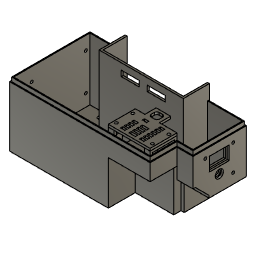
electronics_case (Autodesk Fusion 360 design; units mm, degrees)
Autodesk Fusion 360 part; units mm, degrees
(part 1 of 2)
sketch "Bodenplatte" plane through (0, 0, 0) normal (0, 0, 1) x (1, 0, 0) in component "Boden"
  line L0 (0, 0) -> (123, 0)
  line L1 (175, 42.5) -> (175, 80)
  line L2 (154, 100) -> (0, 100)
  line L3 (0, 100) -> (0, 0)
  line L4 (171, 33.5) -> (123, 33.5)
  line L5 (123, 33.5) -> (123, 0)
  line L6 (154, 100) -> (154, 80)
  line L7 (154, 80) -> (175, 80)
  line L8 (175, 42.5) -> (171, 42.5)
  line L9 (171, 42.5) -> (171, 33.5)
  line L10 (120.5, 20) -> (105.5, 20)
  line L11 (105.5, 20) -> (105.5, 35)
  line L12 (105.5, 35) -> (120.5, 35)
  line L13 (120.5, 35) -> (120.5, 20)
  dimension "d2" = 100
  dimension "d3" = 20
  dimension "d4" = 21
  dimension "d7" = 33
  dimension "d8" = 4
  dimension "d9" = 9
  dimension "d10" = 49
  dimension "d11" = 133.3838
  dimension "d12" = 15
  dimension "d13" = 15
  dimension "d14" = 2.5
  dimension "d76" = 37.5
  dimension "d77" = 52
  dimension "d83" = 20
  dimension "d153" = 175
  constraint horizontal L0
  constraint vertical L1
  constraint horizontal L2
  constraint vertical L3
  constraint coincident L0.start L3.end
  constraint perpendicular L1 L4
  constraint perpendicular L0 L5
  constraint perpendicular L2 L6
  constraint perpendicular L1 L7
  constraint perpendicular L1 L8
  constraint perpendicular L4 L9
  constraint horizontal L10
  constraint vertical L11
  constraint horizontal L12
  constraint vertical L13
  measures "d2" distance of L0.start L2.end
  measures "d3" distance of L2.start L6.end
  measures "d4" distance of L6.end L1.end
  measures "d8" distance of L1.start L8.end
  measures "d9" distance of L8.end L4.start
  measures "d12" distance of L10.start L10.end
  measures "d13" distance of L10.start L12.end
  measures "d14" distance of L5 L13
  measures "d76" distance of L1.end L1.start
  measures "d77" distance of L1 L5
  measures "d83" distance of L0 L10
  measures "d153" distance of L1 L3
extrude "Extrude1" add sketch "Bodenplatte" along normal blind 2.5 makes body 1 in component "Boden"
sketch "Winkel" plane through (0, 100, 0) normal (0, 1, 0) x (-1, 0, 0) in component "Boden"
  line L0 (-154, 0) -> (0, 0)
  line L1 (0, 0) -> (0, 2.5)
  line L2 (0, 2.5) -> (-154, 2.5)
  line L3 (-154, 2.5) -> (-154, 0)
  line L4 (-154, 2.5) -> (-154, 3.5)
  line L5 (-154, 3.5) -> (-170.5, 20)
  line L6 (-170.5, 20) -> (-195, 20)
  line L7 (-195, 20) -> (-195, 22.5)
  line L8 (-195, 22.5) -> (-169.4645, 22.5)
  line L9 (-169.4645, 22.5) -> (-151.5, 4.5355)
  line L10 (-151.5, 4.5355) -> (-151.5, 2.5)
  line L11 (-175, 0) -> (-175, 2.5)
  line L12 (-123, 2.5) -> (-171, 2.5)
  line L13 (-154, 0) -> (0, 0)
  dimension "d17" = 135
  dimension "d19" = 20.5
  dimension "d20" = 2.5
  dimension "d21" = 2.5
  dimension "d22" = 2.5
  dimension "d24" = 20
  dimension "d44" = 3.5
  dimension "d45" = 4.5
  constraint coincident L2.end L3.start
  constraint perpendicular L2 L4
  constraint horizontal L6
  constraint perpendicular L6 L7
  constraint perpendicular L7 L8
  constraint parallel L5 L9
  constraint coincident L2 L10.end
  constraint perpendicular L2 L10
  measures "d17" angle of L4 L5
  measures "d20" distance of L6.end L7.end
  measures "d21" distance of L5 L9
  measures "d22" distance of L4 L10
  measures "d24" distance of L7 L11
  measures "d44" distance of L4.end L13
  measures "d45" distance of L5.end L11
extrude "Extrude6" add sketch "Winkel" against normal up to surface (20 mm away) contours L2 L4 L5 L6 L7 L8 L9 L10 L12 bodies 1 in component "Boden"
sketch "Winkelabdeckung" plane through (0, 80, 0) normal (0, -1, 0) x (1, 0, 0) in component "Boden"
  line L0 (195, 22.5) -> (169.4645, 22.5)
  line L1 (169.4645, 22.5) -> (151.5, 4.5355)
  line L2 (151.5, 4.5355) -> (151.5, 2.5)
  line L3 (151.5, 2.5) -> (154, 2.5)
  line L4 (154, 2.5) -> (154, 3.5) construction
  line L5 (154, 3.5) -> (170.5, 20) construction
  line L6 (170.5, 20) -> (195, 20) construction
  line L7 (195, 20) -> (195, 22.5)
  line L8 (151.5, 2.5) -> (151.5, 4.5355)
  line L9 (151.5, 4.5355) -> (169.4645, 22.5)
  line L10 (186.3838, 2.5) -> (151.5, 2.5)
  line L11 (175, 0) -> (175, 2.5)
  line L12 (175, 2.5) -> (175, 20)
  line L13 (175, 20) -> (195, 20)
  line L14 (195, 20) -> (195, 22.5)
  line L15 (195, 22.5) -> (169.4645, 22.5)
  constraint coincident L2.end L3.start
  constraint coincident L1.end L2.start
  constraint coincident L0.end L1.start
  constraint perpendicular L8 L10
  constraint coincident L11.end L12.start
  constraint coincident L6 L12.end
  constraint perpendicular L6 L12
  constraint coincident L6.end L7.start
  constraint coincident L0.start L7.end
extrude "Extrude7" add sketch "Winkelabdeckung" along normal blind 2.5 bodies 1 in component "Boden"
sketch "Stangenabdeckung" plane through (0, 77.5, 0) normal (0, -1, 0) x (1, 0, 0) in component "Boden"
  line L0 (175, 2.5) -> (175, 20)
  line L1 (175, 20) -> (195, 20)
  line L2 (195, 20) -> (195, 22.5)
  line L3 (195, 22.5) -> (169.4645, 22.5)
  line L4 (169.4645, 22.5) -> (151.5, 4.5355)
  line L5 (151.5, 4.5355) -> (151.5, 2.5)
  line L6 (151.5, 2.5) -> (175, 2.5)
  line L7 (175, 20) -> (195, 20)
  line L8 (195, 20) -> (195, 22.5)
  line L9 (195, 22.5) -> (172.5, 22.5)
  line L10 (172.5, 22.5) -> (172.5, 2.5)
  line L11 (172.5, 2.5) -> (175, 2.5)
  line L12 (175, 2.5) -> (175, 20)
  dimension "d50" = 2.5
  constraint coincident L0.end L1.start
  constraint coincident L1.end L2.start
  constraint coincident L2.end L3.start
  constraint coincident L3 L9.end
  constraint perpendicular L8 L9
  constraint coincident L6 L10.end
  constraint perpendicular L6 L10
  constraint coincident L0.start L6.end
  measures "d50" distance of L10 L12
extrude "Extrude8" add sketch "Stangenabdeckung" along normal blind 26.5 from surface at -2.5 contours L0 L1 L2 L3 L6 L7 L8 L9 L10 L11 L12 bodies 1 in component "Boden"
sketch "Seitenwinkel" plane through (195, 0, 0) normal (1, 0, 0) x (0, 1, 0) in component "Boden"
  line L0 (53.5, 20) -> (100, 20)
  line L1 (100, 20) -> (100, 22.5)
  line L2 (100, 22.5) -> (53.5, 22.5)
  line L3 (53.5, 22.5) -> (53.5, 20)
  line L4 (53.5, 22.5) -> (53.5, 23)
  line L5 (53.5, 23) -> (36.5, 40)
  line L6 (37.5355, 42.5) -> (56, 24.0355)
  line L7 (56, 24.0355) -> (56, 22.5)
  line L8 (36.5, 40) -> (33.5, 40)
  line L9 (33.5, 40) -> (33.5, 42.5)
  line L10 (33.5, 42.5) -> (37.5355, 42.5)
  dimension "d54" = 135
  dimension "d56" = 2.5
  dimension "d57" = 2.5
  dimension "d58" = 2.5
  dimension "d60" = 3
  dimension "d61" = 3
  dimension "d62" = 20
  dimension "d63" = 20
  constraint coincident L2.end L3.start
  constraint perpendicular L2 L4
  constraint parallel L5 L6
  constraint coincident L2 L7.end
  constraint perpendicular L2 L7
  constraint horizontal L8
  constraint perpendicular L8 L9
  constraint perpendicular L9 L10
  measures "d54" angle of L4 L5
  measures "d56" distance of L4 L7
  measures "d57" distance of L5 L6
  measures "d58" distance of L8.end L9.end
  measures "d60" distance of L5.end L8.end
  measures "d61" distance of L0 L4.end
  measures "d62" distance of L3 L9
  measures "d63" distance of L0 L8
extrude "Extrude9" add sketch "Seitenwinkel" against normal up to surface (20 mm away) contours L2 L4 L5 L6 L7 L8 L9 L10 bodies 1 in component "Boden"
sketch "Seitenwinkelabdeckung" plane through (175, 0, 0) normal (1, 0, 0) x (0, 1, 0) in component "Boden"
  line L0 (53.5, 2.5) -> (42.5, 2.5)
  line L1 (42.5, 2.5) -> (42.5, 0)
  line L2 (42.5, 0) -> (80, 0)
  line L3 (80, 0) -> (80, 20)
  line L4 (80, 20) -> (53.5, 20)
  line L5 (53.5, 20) -> (53.5, 2.5)
  line L6 (45, 2.5) -> (53.5, 2.5)
  line L7 (45, 35.0355) -> (45, 2.5)
  line L8 (53.5, 23) -> (36.5, 40)
  line L9 (37.5355, 42.5) -> (56, 24.0355)
  line L10 (53.5, 2.5) -> (53.5, 22.5)
  line L11 (53.5, 22.5) -> (56, 22.5)
  line L12 (56, 22.5) -> (56, 24.0355)
  line L13 (56, 24.0355) -> (45, 35.0355)
  line L14 (56, 24.0355) -> (56, 22.5)
  line L15 (77.5, 22.5) -> (53.5, 22.5)
  dimension "d66" = 4
  dimension "d70" = 2.5
  constraint coincident L0.start L5.end
  constraint perpendicular L6 L7
  constraint perpendicular L6 L10
  constraint perpendicular L10 L11
  constraint collinear L9 L13
  constraint collinear L12 L14
  constraint collinear L11 L15
  measures "d70" distance of L1 L7
extrude "Extrude10" add sketch "Seitenwinkelabdeckung" against normal up to surface (2.5 mm away) contours L0 L5 L6 L7 L9 L10 L11 L12 L13 L14 L15 bodies 1 in component "Boden"
sketch "Sketch8" plane through (0, 0, 2.5) normal (0, 0, 1) x (-1, 0, 0) in component "Boden"
  line L0 (-105.5, -35) -> (-120.5, -35)
  line L1 (-120.5, -35) -> (-120.5, -20)
  line L2 (-120.5, -20) -> (-105.5, -20)
  line L3 (-105.5, -20) -> (-105.5, -35)
  line L4 (-175, -45) -> (-172.5, -45)
  line L5 (-172.5, -45) -> (-172.5, -77.5)
  line L6 (-172.5, -77.5) -> (-151.5, -77.5)
  line L7 (-151.5, -77.5) -> (-151.5, -100)
  line L8 (-151.5, -100) -> (0, -100)
  line L9 (0, -100) -> (0, 0)
  line L10 (0, 0) -> (-123, 0)
  line L11 (-123, 0) -> (-123, -33.5)
  line L12 (-123, -33.5) -> (-171, -33.5)
  line L13 (-171, -33.5) -> (-171, -42.5)
  line L14 (-171, -42.5) -> (-175, -42.5)
  line L15 (-175, -42.5) -> (-175, -45)
  line L16 (-172.5, -45) -> (-168.5, -45)
  line L17 (-168.5, -45) -> (-168.5, -33.5)
  dimension "d71" = 2.5
  constraint coincident L4.end L5.start
  constraint perpendicular L5 L16
  constraint coincident L12 L17.end
  constraint perpendicular L12 L17
  measures "d71" distance of L13 L17
extrude "Extrude11" add sketch "Sketch8" along normal up to surface (52 mm away) contours L4 L12 L13 L14 L15 L16 L17 bodies 1 in component "Boden"
sketch "Sketch9" plane through (175, 0, 0) normal (-1, 0, 0) x (0, -1, 0) in component "Boden"
  line L0 (-42.5, 37.5355) -> (-42.5, 34)
  line L1 (-42.5, 34) -> (-36.5, 40)
  line L2 (-36.5, 40) -> (-33.5, 40)
  line L3 (-33.5, 40) -> (-33.5, 42.5)
  line L4 (-33.5, 42.5) -> (-37.5355, 42.5)
  line L5 (-37.5355, 42.5) -> (-42.5, 37.5355)
  line L6 (-45, 35.0355) -> (-45, 54.5)
  line L7 (-45, 54.5) -> (-33.5, 54.5)
  line L8 (-33.5, 54.5) -> (-33.5, 42.5)
  line L9 (-37.5355, 42.5) -> (-45, 35.0355)
  line L10 (-45, 35.0355) -> (-45, 54.5)
  line L11 (-33.5, 42.5) -> (-37.5355, 42.5)
  line L12 (-45, 54.5) -> (-42.5, 54.5)
  constraint vertical L6
  constraint perpendicular L6 L7
  constraint coincident L4 L3.end
  constraint perpendicular L4 L8
  constraint coincident L4.end L5.start
  constraint collinear L3 L8
  constraint collinear L6 L10
  constraint collinear L5 L9
  constraint collinear L7 L12
extrude "Extrude12" add sketch "Sketch9" against normal blind 2.5 contours L4 L5 L6 L7 L8 L9 L10 L11 L12 bodies 1 in component "Boden"
sketch "Sketch11" plane through (0, 0, 42.5) normal (0, 0, 1) x (-1, 0, 0) in component "Boden"
  line L0 (-177.5, -37.5355) -> (-177.5, -33.5)
  line L1 (-177.5, -33.5) -> (-195, -33.5)
  line L2 (-195, -33.5) -> (-195, -37.5355)
  line L3 (-195, -37.5355) -> (-177.5, -37.5355)
  line L4 (-177.5, -33.5) -> (-195, -33.5)
  line L5 (-195, -33.5) -> (-195, -36)
  line L6 (-195, -36) -> (-177.5, -36)
  line L7 (-177.5, -36) -> (-177.5, -33.5)
  dimension "d78" = 2.5
  constraint horizontal L4
  constraint vertical L5
  constraint horizontal L6
  constraint vertical L7
  constraint coincident L2 L5.end
  constraint coincident L0.end L1.start
  measures "d78" distance of L1.end L5.end
extrude "Extrude13" add sketch "Sketch11" along normal up to surface (12 mm away) contours L0 L1 L2 L4 L5 L6 L7 bodies 1 in component "Boden"
sketch "Sketch12" plane through (195, 0, 0) normal (1, 0, 0) x (0, 1, 0) in component "Boden"
  line L0 (53.5, 20) -> (100, 20)
  line L1 (100, 20) -> (100, 22.5)
  line L2 (100, 22.5) -> (56, 22.5)
  line L3 (56, 22.5) -> (56, 24.0355)
  line L4 (56, 24.0355) -> (37.5355, 42.5)
  line L5 (37.5355, 42.5) -> (36, 42.5)
  line L6 (36, 42.5) -> (36, 54.5)
  line L7 (36, 54.5) -> (33.5, 54.5)
  line L8 (33.5, 54.5) -> (33.5, 40)
  line L9 (33.5, 40) -> (36.5, 40)
  line L10 (36.5, 40) -> (53.5, 23)
  line L11 (53.5, 23) -> (53.5, 20)
  line L12 (100, 22.5) -> (56, 22.5)
  line L13 (56, 24.0355) -> (37.5355, 42.5)
  line L14 (36, 42.5) -> (36, 54.5)
  line L15 (37.5355, 42.5) -> (36, 42.5)
  line L16 (36, 54.5) -> (100, 54.5)
  line L17 (100, 54.5) -> (100, 22.5)
  constraint coincident L1.end L2.start
  constraint coincident L2.end L3.start
  constraint coincident L3.end L4.start
  constraint coincident L4.end L5.start
  constraint coincident L5.end L6.start
  constraint coincident L6.end L7.start
  constraint perpendicular L14 L16
  constraint perpendicular L16 L17
extrude "Extrude14" add sketch "Sketch12" against normal blind 2.5 contours L2 L3 L4 L5 L6 L12 L13 L14 L15 L16 L17 bodies 1 in component "Boden"
sketch "Sketch13" plane through (0, 0, 2.5) normal (0, 0, 1) x (-1, 0, 0) in component "Boden"
  line L0 (-168.5, -33.5) -> (-168.5, -45)
  line L1 (-168.5, -45) -> (-172.5, -45)
  line L2 (-172.5, -45) -> (-172.5, -77.5)
  line L3 (-172.5, -77.5) -> (-151.5, -77.5)
  line L4 (-151.5, -77.5) -> (-151.5, -100)
  line L5 (-151.5, -100) -> (0, -100)
  line L6 (0, -100) -> (0, 0)
  line L7 (0, 0) -> (-123, 0)
  line L8 (-123, 0) -> (-123, -33.5)
  line L9 (-123, -33.5) -> (-168.5, -33.5)
  line L10 (-105.5, -35) -> (-120.5, -35)
  line L11 (-120.5, -35) -> (-120.5, -20)
  line L12 (-120.5, -20) -> (-105.5, -20)
  line L13 (-105.5, -20) -> (-105.5, -35)
  line L14 (-168.5, -36) -> (-120.5, -36)
  line L15 (-120.5, -36) -> (-120.5, -20)
  line L16 (-120.5, -20) -> (-105.5, -20)
  line L17 (-105.5, -20) -> (-105.5, -35)
  line L18 (-105.5, -35) -> (-103, -35)
  line L19 (-103, -35) -> (-103, -17.5)
  line L20 (-103, -17.5) -> (-120.5, -17.5)
  line L21 (-120.5, -17.5) -> (-120.5, 0)
  line L22 (-192.5, -36) -> (-177.5, -36)
  dimension "d84" = 2.5
  dimension "d85" = 2.5
  constraint coincident L0 L14.start
  constraint perpendicular L0 L14
  constraint perpendicular L14 L15
  constraint perpendicular L15 L16
  constraint perpendicular L10 L17
  constraint perpendicular L17 L18
  constraint perpendicular L18 L19
  constraint perpendicular L19 L20
  constraint coincident L7 L21.end
  constraint perpendicular L7 L21
  constraint collinear L11 L15
  constraint collinear L12 L16
  constraint collinear L13 L17
  constraint collinear L10 L18
  constraint collinear L15 L21
  constraint collinear L14 L22
  measures "d84" distance of L17 L19
  measures "d85" distance of L16 L20
extrude "Extrude15" add sketch "Sketch13" along normal up to surface (52 mm away) contours L0 L7 L8 L9 L11 L12 L13 L14 L15 L16 L17 L18 L19 L20 L21 bodies 1 in component "Boden"
sketch "Sketch1" plane through (192.5, 0, 0) normal (-1, 0, 0) x (0, -1, 0) in component "Stromanschluss"
  line L0 (-36, 54.5) -> (-100, 54.5) construction
  line L1 (-100, 54.5) -> (-100, 22.5)
  line L2 (-100, 22.5) -> (-56, 22.5)
  line L3 (-56, 22.5) -> (-56, 24.0355)
  line L4 (-56, 24.0355) -> (-37.5355, 42.5)
  line L5 (-37.5355, 42.5) -> (-36, 42.5)
  line L6 (-36, 42.5) -> (-36, 54.5)
  line L7 (-76.6, 63) -> (-56, 63)
  line L8 (-56, 63) -> (-56, 50)
  line L9 (-56, 50) -> (-76.6, 50)
  line L10 (-76.6, 50) -> (-76.6, 63)
  circle A0 centre (-66.3, 39.75) radius 3.65
  circle A1 centre (-66.3, 39.75) radius 5.25
  line L11 (-76.6, 50) -> (-56, 63) construction
  line L12 (-76.6, 63) -> (-56, 50) construction
  line L13 (-88.6, 70) -> (-44, 70)
  line L14 (-44, 70) -> (-44, 42.5)
  line L15 (-59, 27.5) -> (-88.6, 27.5)
  line L16 (-88.6, 27.5) -> (-88.6, 70)
  line L17 (-59, 27.5) -> (-44, 42.5)
  circle A2 centre (-83.6, 32.5) radius 1.75
  circle A3 centre (-83.6, 65) radius 1.75
  circle A4 centre (-49, 65) radius 1.75
  point P0 (-66.3, 56.5)
  dimension "d91" = 20.6
  dimension "d92" = 13
  dimension "d93" = 7.3
  dimension "d94" = 10.5
  dimension "d95" = 5
  dimension "d96" = 7
  dimension "d97" = 7
  dimension "d98" = 12
  dimension "d99" = 12
  dimension "d105" = 135
  dimension "d106" = 15
  dimension "d107" = 5
  dimension "d108" = 8
  dimension "d113" = 3.5
  dimension "d114" = 5
  dimension "d115" = 5
  dimension "d116" = 5
  dimension "d117" = 5
  constraint horizontal L7
  constraint vertical L8
  constraint horizontal L9
  constraint vertical L10
  constraint concentric A0 A1
  constraint midpoint L12 P0
  constraint vertical A0.centre P0
  constraint horizontal L13
  constraint vertical L14
  constraint horizontal L15
  constraint vertical L16
  constraint vertical A2.centre A3.centre
  constraint horizontal A3.centre A4.centre
  constraint equal A2 A3
  constraint equal A2 A4
  measures "d91" distance of L7.start L7.end
  measures "d92" distance of L7.start L9.end
  measures "d93" diameter of A0
  measures "d94" diameter of A1
  measures "d95" distance of L9 A1
  measures "d96" distance of A1 L15
  measures "d97" distance of L7 L13
  measures "d98" distance of L10 L16
  measures "d99" distance of L8 L14
  measures "d105" angle of L15 L17
  measures "d106" vertical distance of L15.start L14.end
  measures "d107" distance of L2 L15
  measures "d108" distance of L6 L14
  measures "d113" diameter of A2
  measures "d114" distance of L15 A2.centre
  measures "d115" distance of L16 A2.centre
  measures "d116" distance of L13 A3.centre
  measures "d117" distance of L14 A4.centre
sketch "Sketch15" plane through (0, 100, 0) normal (0, 1, 0) x (-1, 0, 0) in component "Boden"
  line L0 (-154, 0) -> (0, 0)
  line L1 (0, 0) -> (0, 2.5)
  line L2 (0, 2.5) -> (-151.5, 2.5)
  line L3 (-151.5, 2.5) -> (-151.5, 4.5355)
  line L4 (-151.5, 4.5355) -> (-169.4645, 22.5)
  line L5 (-169.4645, 22.5) -> (-192.5, 22.5)
  line L6 (-192.5, 22.5) -> (-192.5, 54.5)
  line L7 (-192.5, 54.5) -> (-195, 54.5)
  line L8 (-195, 54.5) -> (-195, 20)
  line L9 (-195, 20) -> (-170.5, 20)
  line L10 (-170.5, 20) -> (-154, 3.5)
  line L11 (-154, 3.5) -> (-154, 0)
  line L12 (-192.5, 54.5) -> (-192.5, 22.5)
  line L13 (-192.5, 22.5) -> (-169.4645, 22.5)
  line L14 (-169.4645, 22.5) -> (-151.5, 4.5355)
  line L15 (-151.5, 4.5355) -> (-151.5, 2.5)
  line L16 (-151.5, 2.5) -> (-146.5, 2.5)
  line L17 (-146.5, 2.5) -> (-146.5, 54.5)
  line L18 (-146.5, 54.5) -> (-192.5, 54.5)
  dimension "d102" = 5
  constraint coincident L6.end L7.start
  constraint coincident L5.end L6.start
  constraint coincident L4.end L5.start
  constraint coincident L3.end L4.start
  constraint coincident L2.end L3.start
  constraint coincident L2 L16.end
  constraint perpendicular L3 L16
  constraint perpendicular L16 L17
  constraint perpendicular L17 L18
  measures "d102" distance of L2.end L16.end
extrude "Extrude17" add sketch "Sketch15" against normal blind 2.5 contours L2 L3 L4 L5 L6 L12 L13 L14 L15 L16 L17 L18 bodies 1 in component "Boden"
extrude "Extrude1'" add sketch "Sketch1" along normal blind 2.5 separate body contours L13 L14 L15 L16 L17 makes body 2 in component "Stromanschluss"
extrude "Extrude2" add sketch "Sketch1" along normal blind 2 contours A1 bodies 2 in component "Stromanschluss"
sketch "Sketch17" plane through (0, 0, 54.5) normal (0, 0, 1) x (-1, 0, 0) in component "Boden"
  line L0 (-177.5, -45) -> (-168.5, -45)
  line L1 (-168.5, -45) -> (-168.5, -36)
  line L2 (-168.5, -36) -> (-120.5, -36)
  line L3 (-120.5, -36) -> (-120.5, -20)
  line L4 (-120.5, -20) -> (-105.5, -20)
  line L5 (-105.5, -20) -> (-105.5, -35)
  line L6 (-105.5, -35) -> (-103, -35)
  line L7 (-103, -35) -> (-103, -17.5)
  line L8 (-103, -17.5) -> (-120.5, -17.5)
  line L9 (-120.5, -17.5) -> (-120.5, 0)
  line L10 (-120.5, 0) -> (-123, 0)
  line L11 (-123, 0) -> (-123, -33.5)
  line L12 (-123, -33.5) -> (-171, -33.5)
  line L13 (-171, -33.5) -> (-171, -42.5)
  line L14 (-171, -42.5) -> (-175, -42.5)
  line L15 (-175, -42.5) -> (-175, -33.5)
  line L16 (-175, -33.5) -> (-195, -33.5)
  line L17 (-195, -33.5) -> (-195, -100)
  line L18 (-195, -100) -> (-146.5, -100)
  line L19 (-146.5, -100) -> (-146.5, -97.5)
  line L20 (-146.5, -97.5) -> (-192.5, -97.5)
  line L21 (-192.5, -97.5) -> (-192.5, -36)
  line L22 (-192.5, -36) -> (-177.5, -36)
  line L23 (-177.5, -36) -> (-177.5, -45)
  line L24 (-123, 0) -> (-175, 0)
  line L25 (-175, 0) -> (-175, -33.5)
  constraint coincident L10.end L11.start
  constraint perpendicular L11 L24
  constraint coincident L12 L15.end
  constraint perpendicular L12 L25
  constraint collinear L15 L25
extrude "Extrude18" add sketch "Sketch17" along normal blind 2.5 bodies 1 in component "Boden"
sketch "Sketch18" plane through (0, 0, 2.5) normal (0, 0, 1) x (-1, 0, 0) in component "Boden"
  line L0 (-146.5, -97.5) -> (-146.5, -100)
  line L1 (-146.5, -100) -> (0, -100)
  line L2 (0, -100) -> (0, 0)
  line L3 (0, 0) -> (-120.5, 0)
  line L4 (-120.5, 0) -> (-120.5, -17.5)
  line L5 (-120.5, -17.5) -> (-103, -17.5)
  line L6 (-103, -17.5) -> (-103, -35)
  line L7 (-103, -35) -> (-105.5, -35)
  line L8 (-105.5, -35) -> (-120.5, -35)
  line L9 (-120.5, -35) -> (-120.5, -36)
  line L10 (-120.5, -36) -> (-168.5, -36)
  line L11 (-168.5, -36) -> (-168.5, -45)
  line L12 (-168.5, -45) -> (-172.5, -45)
  line L13 (-172.5, -45) -> (-172.5, -77.5)
  line L14 (-172.5, -77.5) -> (-151.5, -77.5)
  line L15 (-151.5, -77.5) -> (-151.5, -97.5)
  line L16 (-151.5, -97.5) -> (-146.5, -97.5)
  line L17 (-163.5, -41) -> (-153.5, -41)
  line L18 (-153.5, -41) -> (-153.5, -51)
  line L19 (-153.5, -51) -> (-163.5, -51)
  line L20 (-163.5, -51) -> (-163.5, -41)
  dimension "d120" = 10
  dimension "d121" = 10
  dimension "d122" = 5
  dimension "d123" = 5
  constraint horizontal L17
  constraint vertical L18
  constraint horizontal L19
  constraint vertical L20
  measures "d120" distance of L17.start L17.end
  measures "d121" distance of L17.start L19.end
  measures "d122" distance of L10 L17
  measures "d123" distance of L11 L20
extrude "Extrude19" cut sketch "Sketch18" against normal up to surface (2.5 mm away) contours L17 L18 L19 L20 bodies 1 in component "Boden"
sketch "Sketch19" plane through (0, 0, 2.5) normal (0, 0, 1) x (-1, 0, 0) in component "Boden"
  line L0 (-163.5, -51) -> (-163.5, -41)
  line L1 (-163.5, -41) -> (-153.5, -41)
  line L2 (-153.5, -41) -> (-153.5, -51)
  line L3 (-153.5, -51) -> (-163.5, -51)
  line L4 (-146.5, -97.5) -> (-146.5, -100)
  line L5 (-146.5, -100) -> (0, -100)
  line L6 (0, -100) -> (0, 0)
  line L7 (0, 0) -> (-120.5, 0)
  line L8 (-120.5, 0) -> (-120.5, -17.5)
  line L9 (-120.5, -17.5) -> (-103, -17.5)
  line L10 (-103, -17.5) -> (-103, -35)
  line L11 (-103, -35) -> (-105.5, -35)
  line L12 (-105.5, -35) -> (-120.5, -35)
  line L13 (-120.5, -35) -> (-120.5, -36)
  line L14 (-120.5, -36) -> (-168.5, -36)
  line L15 (-168.5, -36) -> (-168.5, -45)
  line L16 (-168.5, -45) -> (-172.5, -45)
  line L17 (-172.5, -45) -> (-172.5, -77.5)
  line L18 (-172.5, -77.5) -> (-151.5, -77.5)
  line L19 (-151.5, -77.5) -> (-151.5, -97.5)
  line L20 (-151.5, -97.5) -> (-146.5, -97.5)
  line L21 (-146.5, -97.5) -> (-146.5, -70)
  line L22 (-146.5, -70) -> (-46.5, -70)
  line L23 (-46.5, -70) -> (-46.5, -100)
  line L24 (-44, -100) -> (-44, -67.5)
  line L25 (-44, -67.5) -> (-149, -67.5)
  line L26 (-149, -67.5) -> (-149, -97.5)
  dimension "d126" = 2.5
  dimension "d127" = 2.5
  dimension "d128" = 2.5
  dimension "d129" = 30
  dimension "d130" = 100
  constraint coincident L4.start L20.end
  constraint perpendicular L20 L21
  constraint perpendicular L21 L22
  constraint coincident L5 L23.end
  constraint perpendicular L5 L23
  constraint coincident L5 L24.start
  constraint perpendicular L5 L24
  constraint perpendicular L24 L25
  constraint coincident L20 L26.end
  constraint perpendicular L20 L26
  measures "d126" distance of L21 L26
  measures "d127" distance of L22 L25
  measures "d128" distance of L23 L24
  measures "d129" distance of L22.end L23.end
  measures "d130" distance of L21.end L22.end
extrude "Extrude20" add sketch "Sketch19" along normal blind 5 contours L4 L5 L21 L22 L23 bodies 1 in component "Boden"
extrude "Extrude21" add sketch "Sketch19" along normal up to surface (54.5 mm away) contours L5 L20 L21 L22 L23 L24 L25 L26 bodies 1 in component "Boden"
sketch "Sketch20" plane through (0, 0, 2.5) normal (0, 0, 1) x (-1, 0, 0) in component "Boden"
  line L0 (-163.5, -51) -> (-163.5, -41)
  line L1 (-163.5, -41) -> (-153.5, -41)
  line L2 (-153.5, -41) -> (-153.5, -51)
  line L3 (-153.5, -51) -> (-163.5, -51)
  line L4 (-149, -97.5) -> (-149, -67.5)
  line L5 (-149, -67.5) -> (-44, -67.5)
  line L6 (-44, -67.5) -> (-44, -100)
  line L7 (-44, -100) -> (0, -100)
  line L8 (0, -100) -> (0, 0)
  line L9 (0, 0) -> (-120.5, 0)
  line L10 (-120.5, 0) -> (-120.5, -17.5)
  line L11 (-120.5, -17.5) -> (-103, -17.5)
  line L12 (-103, -17.5) -> (-103, -35)
  line L13 (-103, -35) -> (-105.5, -35)
  line L14 (-105.5, -35) -> (-120.5, -35)
  line L15 (-120.5, -35) -> (-120.5, -36)
  line L16 (-120.5, -36) -> (-168.5, -36)
  line L17 (-168.5, -36) -> (-168.5, -45)
  line L18 (-168.5, -45) -> (-172.5, -45)
  line L19 (-172.5, -45) -> (-172.5, -77.5)
  line L20 (-172.5, -77.5) -> (-151.5, -77.5)
  line L21 (-151.5, -77.5) -> (-151.5, -97.5)
  line L22 (-151.5, -97.5) -> (-149, -97.5)
  line L23 (-107, -17.5) -> (-107, -15.5)
  line L24 (-107, -15.5) -> (-103, -15.5)
  line L25 (-103, -15.5) -> (-103, -13)
  line L26 (-103, -13) -> (-109.5, -13)
  line L27 (-109.5, -13) -> (-109.5, -17.5)
  line L28 (-20, -13) -> (-20, -15.5)
  line L29 (-20, -15.5) -> (-16, -15.5)
  line L30 (-16, -15.5) -> (-16, -17.5)
  line L31 (-16, -17.5) -> (-20, -17.5)
  line L32 (-20, -17.5) -> (-20, -20)
  line L33 (-20, -20) -> (-13.5, -20)
  line L34 (-13.5, -20) -> (-13.5, -13)
  line L35 (-13.5, -13) -> (-20, -13)
  line L36 (-120.5, -20) -> (-105.5, -20)
  line L37 (-103, -15.5) -> (-103, -17.5)
  line L38 (-20, -15.5) -> (-20, -17.5)
  dimension "d135" = 2
  dimension "d136" = 2.5
  dimension "d137" = 2.5
  dimension "d138" = 4
  dimension "d139" = 91
  dimension "d140" = 2
  dimension "d141" = 4
  dimension "d142" = 2.5
  constraint coincident L11 L23.start
  constraint perpendicular L11 L23
  constraint perpendicular L23 L24
  constraint perpendicular L11 L25
  constraint perpendicular L25 L26
  constraint coincident L11 L27.end
  constraint perpendicular L11 L27
  constraint perpendicular L26 L28
  constraint perpendicular L28 L29
  constraint perpendicular L26 L30
  constraint perpendicular L28 L31
  constraint perpendicular L31 L32
  constraint perpendicular L32 L33
  constraint perpendicular L33 L34
  constraint perpendicular L34 L35
  constraint collinear L12 L25
  constraint collinear L11 L31
  constraint collinear L33 L36
  constraint collinear L26 L35
  constraint collinear L28 L32
  constraint coincident L11.end L12.start
  measures "d135" distance of L23.start L23.end
  measures "d136" distance of L24 L26
  measures "d137" distance of L23 L27
  measures "d138" distance of L12 L23
  measures "d139" distance of L23 L30
  measures "d140" distance of L29.end L30.end
  measures "d141" distance of L30.end L31.end
  measures "d142" distance of L30 L34
extrude "Extrude22" add sketch "Sketch20" along normal blind 2.5 contours L11 L23 L24 L25 L26 L27 | L11 L23 L24 L37 | L28 L29 L30 L31 L32 L33 L34 L35 | L29 L30 L31 L38 bodies 1 in component "Boden"
extrude "Extrude23" add sketch "Sketch20" along normal blind 50 from surface at 2.5 contours L11 L23 L24 L25 L26 L27 | L28 L29 L30 L31 L32 L33 L34 L35 bodies 1 in component "Boden"
sketch "Sketch21" plane through (0, 0, 2.5) normal (0, 0, 1) x (-1, 0, 0) in component "Boden"
  line L0 (-20, -13) -> (-13.5, -13)
  line L1 (-13.5, -13) -> (-13.5, -20)
  line L2 (-13.5, -20) -> (-20, -20)
  line L3 (-20, -20) -> (-20, -13)
  line L4 (-109.5, -17.5) -> (-109.5, -13)
  line L5 (-109.5, -13) -> (-103, -13)
  line L6 (-103, -13) -> (-103, -35)
  line L7 (-103, -35) -> (-105.5, -35)
  line L8 (-105.5, -35) -> (-120.5, -35)
  line L9 (-120.5, -35) -> (-120.5, -36)
  line L10 (-120.5, -36) -> (-168.5, -36)
  line L11 (-168.5, -36) -> (-168.5, -45)
  line L12 (-168.5, -45) -> (-172.5, -45)
  line L13 (-172.5, -45) -> (-172.5, -77.5)
  line L14 (-172.5, -77.5) -> (-151.5, -77.5)
  line L15 (-151.5, -77.5) -> (-151.5, -97.5)
  line L16 (-151.5, -97.5) -> (-149, -97.5)
  line L17 (-149, -97.5) -> (-149, -67.5)
  line L18 (-149, -67.5) -> (-44, -67.5)
  line L19 (-44, -67.5) -> (-44, -100)
  line L20 (-44, -100) -> (0, -100)
  line L21 (0, -100) -> (0, 0)
  line L22 (0, 0) -> (-120.5, 0)
  line L23 (-120.5, 0) -> (-120.5, -17.5)
  line L24 (-120.5, -17.5) -> (-109.5, -17.5)
  line L25 (-163.5, -51) -> (-163.5, -41)
  line L26 (-163.5, -41) -> (-153.5, -41)
  line L27 (-153.5, -41) -> (-153.5, -51)
  line L28 (-153.5, -51) -> (-163.5, -51)
  line L29 (-44, -97.5) -> (-2.5, -97.5)
  line L30 (-2.5, -97.5) -> (-2.5, -2.5)
  line L31 (-2.5, -2.5) -> (-120.5, -2.5)
  dimension "d148" = 2.5
  dimension "d150" = 2.5
  dimension "d265" = 2.5
  constraint coincident L19 L29.start
  constraint perpendicular L19 L29
  constraint perpendicular L29 L30
  constraint coincident L23 L31.end
  constraint perpendicular L23 L31
  measures "d148" distance of L20 L29
  measures "d150" distance of L22 L31
  measures "d265" distance of L21 L30
extrude "Extrude24" add sketch "Sketch21" along normal up to surface (54.5 mm away) contours L19 L20 L21 L22 L23 L29 L30 L31 bodies 1 in component "Boden"
sketch "Sketch22" plane through (0, 0, 57) normal (0, 0, 1) x (-1, 0, 0) in component "Boden"
  line L0 (-44, -97.5) -> (-44, -67.5)
  line L1 (-44, -67.5) -> (-149, -67.5)
  line L2 (-149, -67.5) -> (-149, -97.5)
  line L3 (-149, -97.5) -> (-192.5, -97.5)
  line L4 (-192.5, -97.5) -> (-192.5, -36)
  line L5 (-192.5, -36) -> (-177.5, -36)
  line L6 (-177.5, -36) -> (-177.5, -45)
  line L7 (-177.5, -45) -> (-168.5, -45)
  line L8 (-168.5, -45) -> (-168.5, -36)
  line L9 (-168.5, -36) -> (-120.5, -36)
  line L10 (-120.5, -36) -> (-120.5, -20)
  line L11 (-120.5, -20) -> (-105.5, -20)
  line L12 (-105.5, -20) -> (-105.5, -35)
  line L13 (-105.5, -35) -> (-103, -35)
  line L14 (-103, -35) -> (-103, -17.5)
  line L15 (-103, -17.5) -> (-120.5, -17.5)
  line L16 (-120.5, -17.5) -> (-120.5, -2.5)
  line L17 (-120.5, -2.5) -> (-2.5, -2.5)
  line L18 (-46.5, -100) -> (0, -100)
  line L19 (0, 0) -> (-175, 0)
  line L20 (-195, -33.5) -> (-195, -100)
  line L21 (-146.5, -100) -> (-146.5, -70)
  line L22 (-146.5, -70) -> (-46.5, -70)
  line L23 (-46.5, -70) -> (-46.5, -100)
  line L24 (-120.5, -20) -> (-120.5, -17.5)
  line L25 (-172.5, -2.5) -> (-120.5, -2.5)
  line L26 (-2.5, -2.5) -> (-2.5, -97.5)
  line L27 (-2.5, -97.5) -> (-44, -97.5)
  line L28 (0, -100) -> (0, 0)
  line L29 (-195, -100) -> (-146.5, -100)
  line L30 (-175, 0) -> (-175, -33.5)
  line L31 (-175, -33.5) -> (-195, -33.5)
  line L32 (-177.5, -36) -> (-172.5, -36)
  line L33 (-172.5, -36) -> (-172.5, -2.5)
  line L34 (-172.5, -77.5) -> (-172.5, -56)
  constraint coincident L10.end L11.start
  constraint coincident L15.end L16.start
  constraint coincident L16.end L17.start
  constraint perpendicular L16 L25
  constraint coincident L5.end L6.start
  constraint perpendicular L6 L32
  constraint perpendicular L25 L33
  constraint collinear L33 L34
extrude "Extrude26" add sketch "Sketch22" along normal up to surface (18 mm away) bodies 1 in component "Boden"
sketch "Sketch24" plane through (192.5, 0, 0) normal (-1, 0, 0) x (0, -1, 0) in component "Boden"
  line L0 (-97.5, 75) -> (-97.5, 22.5)
  line L1 (-97.5, 22.5) -> (-56, 22.5)
  line L2 (-56, 22.5) -> (-56, 24.0355)
  line L3 (-56, 24.0355) -> (-37.5355, 42.5)
  line L4 (-37.5355, 42.5) -> (-36, 42.5)
  line L5 (-36, 42.5) -> (-36, 75)
  line L6 (-36, 75) -> (-97.5, 75)
  line L7 (-78.6, 65) -> (-54, 65)
  line L8 (-54, 65) -> (-54, 48)
  line L9 (-54, 48) -> (-78.6, 48)
  line L10 (-78.6, 48) -> (-78.6, 65)
  line L11 (-76.6, 63) -> (-56, 63) construction
  line L12 (-56, 63) -> (-56, 50) construction
  line L13 (-56, 50) -> (-76.6, 50) construction
  line L14 (-76.6, 50) -> (-76.6, 63) construction
  circle A0 centre (-66.3, 39.75) radius 5.15
  circle A1 centre (-66.3, 39.75) radius 3.65 construction
  circle A2 centre (-83.6, 32.5) radius 1.75
  circle A3 centre (-83.6, 65) radius 1.75
  circle A4 centre (-49, 65) radius 1.75
  circle A5 centre (-83.6, 32.5) radius 1.75
  circle A6 centre (-83.6, 65) radius 1.75
  circle A7 centre (-49, 65) radius 1.75
  dimension "d158" = 2
  dimension "d159" = 2
  dimension "d160" = 2
  dimension "d161" = 2
  dimension "d163" = 10.3
  constraint horizontal L7
  constraint vertical L8
  constraint horizontal L9
  constraint vertical L10
  constraint concentric A0 A1
  constraint equal A2 A5
  constraint equal A3 A6
  constraint equal A4 A7
  constraint concentric A4 A7
  constraint concentric A3 A6
  constraint concentric A2 A5
  measures "d158" distance of L7 L11
  measures "d159" distance of L8 L12
  measures "d160" distance of L9 L13
  measures "d161" distance of L10 L14
  measures "d163" diameter of A0
extrude "Extrude27" cut sketch "Sketch24" against normal up to surface (2.5 mm away) contours L7 L8 L9 L10 | A0 | A2 A5 | A3 A6 | A4 A7 bodies 1 in component "Boden"
extrude "Extrude28" add sketch "Sketch21" against normal up to surface (2.5 mm away) contours L0 L1 L2 L3 | L4 L5 L6 L7 L8 L9 L10 L11 L12 L13 L14 L15 L16 L17 L18 L19 L23 L24 L29 L30 L31 | L19 L20 L21 L22 L23 L29 L30 L31 | L25 L26 L27 L28 bodies 1 in component "Boden"
sketch "Sketch25" plane through (2.5, 0, 0) normal (1, 0, 0) x (0, 1, 0) in component "Boden"
  line L0 (2.5, 75) -> (2.5, 2.5)
  line L1 (2.5, 2.5) -> (97.5, 2.5)
  line L2 (97.5, 2.5) -> (97.5, 75)
  line L3 (97.5, 75) -> (2.5, 75)
  circle A0 centre (92.5, 63.6) radius 1.75
  circle A1 centre (25, 63.6) radius 1.75
  circle A2 centre (25, 17.5) radius 1.75
  circle A3 centre (92.5, 17.5) radius 1.75
  dimension "d172" = 3.5
  dimension "d173" = 3.5
  dimension "d174" = 64
  dimension "d175" = 42.6
  dimension "d176" = 5
  dimension "d177" = 17.5
  dimension "d178" = 15
  constraint equal A0 A1
  constraint equal A1 A2
  constraint equal A2 A3
  constraint vertical A0.centre A3.centre
  constraint horizontal A2.centre A3.centre
  constraint vertical A1.centre A2.centre
  constraint horizontal A0.centre A1.centre
  measures "d172" diameter of A0
  measures "d173" diameter of A1
  measures "d174" distance of A0 A1
  measures "d175" distance of A0 A3
  measures "d176" distance of L2 A0.centre
  measures "d178" distance of L1 A2.centre
extrude "Extrude30" cut sketch "Sketch25" against normal up to surface (2.5 mm away) contours A0 | A1 | A2 | A3 bodies 1 in component "Boden"
sketch "Sketch26" plane through (0, 0, 75) normal (0, 0, 1) x (-1, 0, 0) in component "Boden"
  line L0 (-172.5, -2.5) -> (-2.5, -2.5)
  line L1 (-2.5, -2.5) -> (-2.5, -97.5)
  line L2 (-2.5, -97.5) -> (-44, -97.5)
  line L3 (-44, -97.5) -> (-44, -67.5)
  line L4 (-44, -67.5) -> (-149, -67.5)
  line L5 (-149, -67.5) -> (-149, -97.5)
  line L6 (-149, -97.5) -> (-192.5, -97.5)
  line L7 (-192.5, -97.5) -> (-192.5, -36)
  line L8 (-46.5, -100) -> (0, -100)
  line L9 (0, 0) -> (-175, 0)
  line L10 (-195, -33.5) -> (-195, -100)
  line L11 (-195, -100) -> (-146.5, -100)
  line L12 (-146.5, -100) -> (-146.5, -70)
  line L13 (-146.5, -70) -> (-46.5, -70)
  line L14 (-46.5, -70) -> (-46.5, -100)
  line L15 (-44, -97.5) -> (-44, -100)
  line L16 (-149, -97.5) -> (-149, -100)
  line L17 (0, -100) -> (0, 0)
  line L18 (-175, -33.5) -> (-195, -33.5)
  line L19 (-175, 0) -> (-175, -33.5)
  line L20 (-172.5, -36) -> (-172.5, -2.5)
  line L21 (-192.5, -36) -> (-172.5, -36)
  constraint coincident L2.end L3.start
  constraint coincident L8 L15.end
  constraint perpendicular L8 L15
  constraint coincident L5.end L6.start
  constraint coincident L11 L16.end
  constraint perpendicular L11 L16
extrude "Extrude31" add sketch "Sketch26" along normal blind 22.5 contours L3 L4 L5 L8 L11 L12 L13 L14 L15 L16 bodies 1 in component "Boden"
sketch "Sketch27" plane through (0, 70, 0) normal (0, 1, 0) x (-1, 0, 0) in component "Boden"
  line L0 (-146.5, 7.5) -> (-46.5, 7.5)
  line L1 (-46.5, 7.5) -> (-46.5, 97.5)
  line L2 (-46.5, 97.5) -> (-146.5, 97.5)
  line L3 (-146.5, 97.5) -> (-146.5, 7.5)
  line L4 (-126.5, 89.5) -> (-104, 89.5)
  line L5 (-104, 89.5) -> (-104, 82.5)
  line L6 (-104, 82.5) -> (-126.5, 82.5)
  line L7 (-126.5, 82.5) -> (-126.5, 89.5)
  line L8 (-94, 89.5) -> (-71.5, 89.5)
  line L9 (-71.5, 89.5) -> (-71.5, 82.5)
  line L10 (-71.5, 82.5) -> (-94, 82.5)
  line L11 (-94, 82.5) -> (-94, 89.5)
  dimension "d183" = 7
  dimension "d184" = 20
  dimension "d185" = 10
  dimension "d186" = 25
  dimension "d187" = 75
  constraint horizontal L4
  constraint vertical L5
  constraint horizontal L6
  constraint vertical L7
  constraint horizontal L8
  constraint vertical L9
  constraint horizontal L10
  constraint vertical L11
  constraint collinear L4 L8
  constraint collinear L6 L10
  constraint equal L4 L8
  measures "d183" distance of L4.start L6.end
  measures "d184" distance of L3 L7
  measures "d185" distance of L5 L11
  measures "d186" distance of L1 L9
  measures "d187" distance of L0 L6
extrude "Extrude32" cut sketch "Sketch27" against normal up to surface (2.5 mm away) contours L4 L5 L6 L7 | L8 L9 L10 L11 bodies 1 in component "Boden"
sketch "Sketch28" plane through (0, 0, 57) normal (0, 0, 1) x (-1, 0, 0) in component "Boden"
  line L0 (-120.5, -2.5) -> (-172.5, -2.5)
  line L1 (-172.5, -36) -> (-177.5, -36)
  line L2 (-177.5, -36) -> (-177.5, -45)
  line L3 (-177.5, -45) -> (-168.5, -45)
  line L4 (-168.5, -45) -> (-168.5, -36)
  line L5 (-168.5, -36) -> (-120.5, -36)
  line L6 (-120.5, -36) -> (-120.5, -20)
  line L7 (-120.5, -20) -> (-105.5, -20)
  line L8 (-105.5, -20) -> (-105.5, -35)
  line L9 (-105.5, -35) -> (-103, -35)
  line L10 (-103, -35) -> (-103, -17.5)
  line L11 (-103, -17.5) -> (-120.5, -17.5)
  line L12 (-120.5, -17.5) -> (-120.5, -2.5)
  line L13 (-120.5, -36) -> (-127.5, -36)
  line L14 (-127.5, -36) -> (-127.5, -33)
  line L15 (-127.5, -33) -> (-120.5, -33)
  line L16 (-120.5, -33) -> (-120.5, -36)
  line L17 (-120.5, -2.5) -> (-127.5, -2.5)
  line L18 (-127.5, -2.5) -> (-127.5, -5.5)
  line L19 (-127.5, -5.5) -> (-120.5, -5.5)
  line L20 (-120.5, -5.5) -> (-120.5, -2.5)
  line L21 (-172.5, -36) -> (-165.5, -36)
  line L22 (-165.5, -36) -> (-165.5, -33)
  line L23 (-165.5, -33) -> (-172.5, -33)
  line L24 (-172.5, -33) -> (-172.5, -36)
  line L25 (-172.5, -2.5) -> (-172.5, -36)
  line L26 (-165.5, -2.5) -> (-172.5, -2.5)
  line L27 (-172.5, -2.5) -> (-172.5, -5.5)
  line L28 (-172.5, -5.5) -> (-165.5, -5.5)
  line L29 (-165.5, -5.5) -> (-165.5, -2.5)
  dimension "d190" = 3
  dimension "d191" = 7
  dimension "d192" = 3
  dimension "d193" = 7
  dimension "d194" = 3
  dimension "d196" = 7
  constraint horizontal L13
  constraint vertical L14
  constraint horizontal L15
  constraint vertical L16
  constraint coincident L5.end L6.start
  constraint horizontal L17
  constraint vertical L18
  constraint horizontal L19
  constraint vertical L20
  constraint coincident L0.start L12.end
  constraint horizontal L21
  constraint vertical L22
  constraint horizontal L23
  constraint vertical L24
  constraint coincident L1.start L21.start
  constraint horizontal L26
  constraint vertical L27
  constraint horizontal L28
  constraint vertical L29
  constraint coincident L25 L27.end
  constraint coincident L0 L26.start
  constraint collinear L19 L28
  constraint collinear L22 L29
  measures "d190" distance of L5.end L15.end
  measures "d191" distance of L5.end L13.end
  measures "d192" distance of L0.start L19.end
  measures "d193" distance of L0.start L17.end
  measures "d194" distance of L1.start L23.end
  measures "d196" distance of L1.start L21.end
extrude "Extrude33" add sketch "Sketch28" along normal blind 25 contours L0 L12 L17 L18 L19 L20 | L0 L25 L26 L27 L28 L29 | L5 L21 L22 L23 L24 L25 | L5 L6 L13 L14 L15 L16 bodies 1 in component "Boden"
sketch "Sketch29" plane through (0, 0, 82) normal (0, 0, 1) x (-1, 0, 0) in component "Boden"
  line L0 (-120.5, -36) -> (-127.5, -36)
  line L1 (-127.5, -36) -> (-127.5, -2.5)
  line L2 (-127.5, -2.5) -> (-120.5, -2.5)
  line L3 (-120.5, -2.5) -> (-120.5, -36)
  line L4 (-165.5, -36) -> (-172.5, -36)
  line L5 (-172.5, -36) -> (-172.5, -2.5)
  line L6 (-172.5, -2.5) -> (-165.5, -2.5)
  line L7 (-165.5, -2.5) -> (-165.5, -36)
  line L8 (-165.5, -2.5) -> (-172.5, -2.5)
  line L9 (-172.5, -36) -> (-165.5, -36)
  line L10 (-172.5, -33) -> (-172.5, -36)
  line L11 (-165.5, -36) -> (-165.5, -33)
  line L12 (-120.5, -2.5) -> (-127.5, -2.5)
  line L13 (-120.5, -5.5) -> (-120.5, -2.5)
  line L14 (-127.5, -2.5) -> (-127.5, -5.5)
  line L15 (-127.5, -36) -> (-120.5, -36)
  constraint horizontal L0
  constraint vertical L1
  constraint horizontal L2
  constraint vertical L3
  constraint horizontal L4
  constraint vertical L5
  constraint horizontal L6
  constraint vertical L7
  constraint collinear L6 L8
  constraint collinear L4 L9
  constraint collinear L5 L10
  constraint collinear L7 L11
  constraint collinear L2 L12
  constraint collinear L3 L13
  constraint collinear L1 L14
  constraint collinear L0 L15
extrude "Extrude34" add sketch "Sketch29" along normal blind 3 bodies 1 in component "Boden"
sketch "Sketch31" plane through (0, 0, 75) normal (0, 0, 1) x (-1, 0, 0) in component "Boden"
  line L0 (-165.5, -2.5) -> (-127.5, -2.5)
  line L1 (-127.5, -2.5) -> (-120.5, -2.5)
  line L2 (-120.5, -2.5) -> (-2.5, -2.5)
  line L3 (-2.5, -2.5) -> (-2.5, -97.5)
  line L4 (-2.5, -97.5) -> (-44, -97.5)
  line L5 (-44, -100) -> (0, -100)
  line L6 (0, 0) -> (-175, 0)
  line L7 (-149, -98.75) -> (-149, -97.5)
  line L8 (-44, -98.75) -> (-44, -97.5)
  line L9 (0, -100) -> (0, 0)
  line L10 (-175, 0) -> (-175, -33.5)
  line L11 (-192.5, -36) -> (-172.5, -36)
  line L12 (-172.5, -36) -> (-172.5, -33)
  line L13 (-172.5, -33) -> (-172.5, -5.5)
  line L14 (-172.5, -2.5) -> (-165.5, -2.5)
  line L15 (-149, -97.5) -> (-192.5, -97.5)
  line L16 (-192.5, -97.5) -> (-192.5, -36)
  line L17 (-195, -33.5) -> (-195, -100)
  line L18 (-195, -100) -> (-149, -100)
  line L19 (-172.5, -5.5) -> (-172.5, -2.5)
  line L20 (-175, -33.5) -> (-195, -33.5)
  line L21 (-44, -98.75) -> (-1.25, -98.75)
  line L22 (-1.25, -98.75) -> (-1.25, -1.25)
  line L23 (-1.25, -1.25) -> (-173.75, -1.25)
  line L24 (-173.75, -1.25) -> (-173.75, -34.75)
  line L25 (-173.75, -34.75) -> (-193.75, -34.75)
  line L26 (-193.75, -34.75) -> (-193.75, -98.75)
  line L27 (-193.75, -98.75) -> (-149, -98.75)
  dimension "d284" = -1.25
  constraint coincident L4.end L8.end
  constraint perpendicular L4 L8
extrude "Extrude36" add sketch "Sketch31" along normal blind 5 bodies 1 in component "Boden"
sketch "Sketch32" plane through (0, 0, 20) normal (0, 0, -1) x (1, 0, 0) in component "Boden"
  line L0 (175, -80) -> (170.5, -80)
  line L1 (170.5, -80) -> (170.5, -100)
  line L2 (170.5, -100) -> (195, -100)
  line L3 (195, -100) -> (195, -53.5)
  line L4 (195, -53.5) -> (175, -53.5)
  line L5 (175, -53.5) -> (175, -80)
  line L6 (185, -53.5) -> (185, -100) construction
  circle A0 centre (185, -90) radius 2.75
  dimension "d251" = 5.5
  dimension "d252" = 10
  constraint midpoint L4 L6.start
  constraint coincident L2 L6.end
  constraint perpendicular L2 L6
  constraint coincident L6 A0.centre
  measures "d251" diameter of A0
  measures "d252" distance of L2 A0.centre
extrude "Extrude37" cut sketch "Sketch32" against normal up to surface (2.5 mm away) contours A0 bodies 1 in component "Boden"
sketch "Sketch33" plane through (0, 0, 0) normal (0, 0, -1) x (1, 0, 0) in component "Boden"
  line L0 (120.5, -35) -> (105.5, -35)
  line L1 (105.5, -35) -> (105.5, -20)
  line L2 (105.5, -20) -> (120.5, -20)
  line L3 (120.5, -20) -> (120.5, -35)
  line L4 (175, -80) -> (175, -42.5)
  line L5 (175, -42.5) -> (171, -42.5)
  line L6 (171, -42.5) -> (171, -33.5)
  line L7 (171, -33.5) -> (123, -33.5)
  line L8 (123, -33.5) -> (123, 0)
  line L9 (123, 0) -> (0, 0)
  line L10 (0, -100) -> (154, -100)
  line L11 (154, -100) -> (154, -80)
  line L12 (154, -80) -> (175, -80)
  circle A0 centre (83, -10) radius 2.75
  line L13 (0, 0) -> (0, -100)
  dimension "d255" = 5.5
  dimension "d256" = 40
  dimension "d257" = 10
  measures "d255" diameter of A0
  measures "d256" distance of L8 A0.centre
  measures "d257" distance of L9 A0.centre
extrude "Extrude38" cut sketch "Sketch33" against normal up to surface (2.5 mm away) contours A0 bodies 1 in component "Boden"
sketch "Sketch34" plane through (0, 0, 0) normal (0, 0, -1) x (1, 0, 0) in component "Boden"
  circle A0 centre (83, -10) radius 2.75
  line L0 (120.5, -35) -> (105.5, -35)
  line L1 (105.5, -35) -> (105.5, -20)
  line L2 (105.5, -20) -> (120.5, -20)
  line L3 (120.5, -20) -> (120.5, -35)
  line L4 (175, -80) -> (175, -42.5)
  line L5 (175, -42.5) -> (171, -42.5)
  line L6 (171, -42.5) -> (171, -33.5)
  line L7 (171, -33.5) -> (123, -33.5)
  line L8 (123, -33.5) -> (123, 0)
  line L9 (123, 0) -> (0, 0)
  line L10 (0, -100) -> (154, -100)
  line L11 (154, -100) -> (154, -80)
  line L12 (154, -80) -> (175, -80)
  circle A1 centre (22.75, -90) radius 2.75
  line L13 (0, 0) -> (0, -100)
  dimension "d260" = 5.5
  dimension "d261" = 10
  dimension "d276" = 20
  measures "d260" diameter of A1
  measures "d261" distance of L10 A1.centre
  measures "d276" distance of A1 L13
extrude "Extrude39" cut sketch "Sketch34" against normal up to surface (2.5 mm away) contours A1 bodies 1 in component "Boden"
sketch "Sketch35" plane through (0, 0, 7.5) normal (0, 0, 1) x (-1, 0, 0) in component "Boden"
  line L0 (-146.5, -70) -> (-146.5, -100)
  line L1 (-146.5, -100) -> (-46.5, -100)
  line L2 (-46.5, -100) -> (-46.5, -70)
  line L3 (-46.5, -70) -> (-146.5, -70)
  circle A0 centre (-53, -84.65) radius 2.25
  circle A1 centre (-140, -84.65) radius 2.25
  dimension "d266" = 4.5
  dimension "d267" = 82.5
  dimension "d268" = 6.5
  dimension "d269" = 6.8636
  dimension "d270" = 13.1
  constraint equal A0 A1
  constraint horizontal A0.centre A1.centre
  measures "d266" diameter of A0
  measures "d267" distance of A0 A1
  measures "d268" distance of L2 A0.centre
  measures "d270" distance of L1 A0
extrude "Extrude40" cut sketch "Sketch35" against normal up to surface (7.5 mm away) contours A0 | A1 bodies 1 in component "Boden"
sketch "Sketch36" plane through (0, 0, 0) normal (0, 0, -1) x (1, 0, 0) in component "Boden"
  circle A0 centre (140, -84.65) radius 2.25
  circle A1 centre (53, -84.65) radius 2.25
  line L0 (0, 0) -> (0, -100)
  line L1 (0, -100) -> (154, -100)
  line L2 (154, -100) -> (154, -80)
  line L3 (154, -80) -> (175, -80)
  line L4 (175, -80) -> (175, -42.5)
  line L5 (175, -42.5) -> (171, -42.5)
  line L6 (171, -42.5) -> (171, -33.5)
  line L7 (171, -33.5) -> (123, -33.5)
  line L8 (123, -33.5) -> (123, 0)
  line L9 (123, 0) -> (0, 0)
  circle A2 centre (83, -10) radius 2.75
  line L10 (105.5, -35) -> (105.5, -20)
  line L11 (105.5, -20) -> (120.5, -20)
  line L12 (120.5, -20) -> (120.5, -35)
  line L13 (120.5, -35) -> (105.5, -35)
  circle A3 centre (53, -84.65) radius 5.5
  circle A4 centre (140, -84.65) radius 5.5
  circle A5 centre (22.75, -90) radius 2.75
  dimension "d273" = 11
  constraint concentric A1 A3
  constraint concentric A0 A4
  constraint equal A3 A4
  measures "d273" diameter of A3
extrude "Extrude41" cut sketch "Sketch36" against normal up to surface (5.5 mm away) contours A3 | A4 bodies 1 in component "Boden"
sketch "Sketch5" plane through (0, 0, 2.5) normal (0, 0, 1) x (-1, 0, 0) in component "Boden"
  circle A0 centre (-22.75, -90) radius 2.75
  circle A1 centre (-83, -10) radius 2.75
  line L0 (-44, -97.5) -> (-2.5, -97.5)
  line L1 (-2.5, -97.5) -> (-2.5, -2.5)
  line L2 (-2.5, -2.5) -> (-120.5, -2.5)
  line L3 (-120.5, -2.5) -> (-120.5, -17.5)
  line L4 (-120.5, -17.5) -> (-109.5, -17.5)
  line L5 (-109.5, -17.5) -> (-109.5, -13)
  line L6 (-109.5, -13) -> (-103, -13)
  line L7 (-103, -13) -> (-103, -35)
  line L8 (-103, -35) -> (-105.5, -35)
  line L9 (-105.5, -35) -> (-120.5, -35)
  line L10 (-120.5, -35) -> (-120.5, -36)
  line L11 (-120.5, -36) -> (-168.5, -36)
  line L12 (-168.5, -36) -> (-168.5, -45)
  line L13 (-168.5, -45) -> (-172.5, -45)
  line L14 (-172.5, -45) -> (-172.5, -77.5)
  line L15 (-172.5, -77.5) -> (-151.5, -77.5)
  line L16 (-151.5, -77.5) -> (-151.5, -97.5)
  line L17 (-151.5, -97.5) -> (-149, -97.5)
  line L18 (-149, -97.5) -> (-149, -67.5)
  line L19 (-149, -67.5) -> (-44, -67.5)
  line L20 (-44, -67.5) -> (-44, -97.5)
  line L21 (-20, -13) -> (-13.5, -13)
  line L22 (-13.5, -13) -> (-13.5, -20)
  line L23 (-13.5, -20) -> (-20, -20)
  line L24 (-20, -20) -> (-20, -13)
  line L25 (-162.5, -42) -> (-154.5, -42)
  line L26 (-154.5, -42) -> (-154.5, -50)
  line L27 (-154.5, -50) -> (-162.5, -50)
  line L28 (-162.5, -50) -> (-162.5, -42)
  dimension "d277" = 8
  dimension "d278" = 8
  dimension "d279" = 6
  dimension "d280" = 6
  constraint horizontal L25
  constraint vertical L26
  constraint horizontal L27
  constraint vertical L28
  measures "d277" distance of L25.start L25.end
  measures "d278" distance of L25.start L27.end
  measures "d279" distance of L12 L28
  measures "d280" distance of L11 L25
extrude "Extrude42" cut sketch "Sketch5" against normal up to surface (2.5 mm away) contours L25 L26 L27 L28 bodies 1 in component "Boden"